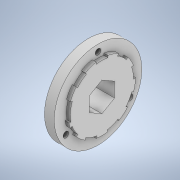
# Autodesk Inventor part: wheel_gearing_mount_short
Saved by Autodesk Inventor 2021 (Build 250183000, 183)
## iProperties
Created: 2021-01-10
Part Number: wheel_gearing_mount_short
Material: Generic
Document SubType Name: Modeling
Designer: Mateusz
Density: 1 g/cm^3
Appearance: Default
Author: Mateusz
Autodesk Inventor part; units mm, degrees
ref_plane "YZ Plane" through (0, 0, 0) normal (1, 0, 0) x (0, 1, 0)
ref_plane "XZ Plane" through (0, 0, 0) normal (0, 1, 0) x (-1, 0, 0)
sketch "Sketch1" plane through (0, 0, 0) normal (1, 0, 0) x (0, 1, 0)
  line L0 (0, 0) -> (7.5, 0)
  line L1 (7.5, 0) -> (3.75, -6.4952)
  line L2 (3.75, -6.4952) -> (-3.75, -6.4952)
  line L3 (-3.75, -6.4952) -> (-7.5, 0)
  line L4 (-7.5, 0) -> (-3.75, 6.4952)
  line L5 (-3.75, 6.4952) -> (3.75, 6.4952)
  line L6 (3.75, 6.4952) -> (7.5, 0)
  circle A0 centre (0, 0) radius 15
  dimension "d0" = 7.5
  dimension "d1" = 30
  constraints: 14 end point, 2 coincident, 1 centre point, 1 horizontal, 13 other
  measures "d0" distance of L0.start L0.end
  measures "d1" diameter of A0
extrude "Extrusion1" add sketch "Sketch1" along normal blind 10.25
sketch "Sketch2" plane through (10.25, 0, 0) normal (1, 0, 0) x (0, 0, -1)
  circle A0 centre (0, 0) radius 22.5
  line L0 (-6.4952, 3.75) -> (0, 7.5) projected
  line L1 (-6.4952, -3.75) -> (-6.4952, 3.75) projected
  line L2 (0, -7.5) -> (-6.4952, -3.75) projected
  line L3 (6.4952, -3.75) -> (0, -7.5) projected
  line L4 (6.4952, 3.75) -> (6.4952, -3.75) projected
  line L5 (0, 7.5) -> (6.4952, 3.75) projected
  dimension "d4" = 45
  constraints: 1 centre point, 1 coincident
  measures "d4" diameter of A0
extrude "Extrusion2" add sketch "Sketch2" against normal blind 5
sketch "Sketch3" plane through (10.25, 0, 0) normal (1, 0, 0) x (0, 0, -1)
  circle A0 centre (0, 19.05) radius 1.45
  circle A1 centre (-16.4978, -9.525) radius 1.45
  circle A2 centre (16.4978, -9.525) radius 1.45
  point P0 (0, 0)
  dimension "d11" = 360
  constraints: 3 centre point, 7 other
extrude "Extrusion3" cut sketch "Sketch3" against normal up to surface (5 mm away)
sketch "Sketch4" plane through (10.25, 0, 0) normal (1, 0, 0) x (0, 0, -1)
  circle A0 centre (0, 19.05) radius 1.45
  line L0 (-3, 17.2409) -> (-3, 16.225)
  line L1 (3, 17.2409) -> (3, 16.225)
  line L2 (13.3804, 11.279) -> (12.7273, 10.5007)
  line L3 (8.7841, 15.1357) -> (8.1311, 14.3574)
  line L4 (17.5, 0.0394) -> (16.4994, -0.137)
  line L5 (16.4581, 5.9483) -> (15.4575, 5.7719)
  line L6 (13.4311, -11.2185) -> (12.5512, -10.7106)
  line L7 (16.4311, -6.0224) -> (15.5512, -5.5144)
  arc A1 (8.7841, 15.1357) -> (3, 17.2409) centre (0, 0) ccw
  arc A2 (16.4311, -6.0224) -> (17.5, 0.0394) centre (0, 0) ccw
  arc A3 (16.4581, 5.9483) -> (13.3804, 11.279) centre (0, 0) ccw
  arc A4 (12.7273, 10.5007) -> (8.1311, 14.3574) centre (0, 0) ccw
  arc A5 (16.4994, -0.137) -> (15.4575, 5.7719) centre (0, 0) ccw
  line L8 (3.0777, -17.2272) -> (2.7302, -16.2726)
  line L9 (3.0777, -17.2272) -> (2.7302, -16.2726)
  line L10 (8.7158, -15.1751) -> (8.3683, -14.2204)
  line L11 (8.7158, -15.1751) -> (8.3683, -14.2204)
  line L12 (-8.7158, -15.1751) -> (-8.3683, -14.2204)
  line L13 (-8.7158, -15.1751) -> (-8.3683, -14.2204)
  line L14 (-3.0777, -17.2272) -> (-2.7302, -16.2726)
  line L15 (-3.0777, -17.2272) -> (-2.7302, -16.2726)
  line L16 (-16.4311, -6.0224) -> (-15.5512, -5.5144)
  line L17 (-16.4311, -6.0224) -> (-15.5512, -5.5144)
  line L18 (-13.4311, -11.2185) -> (-12.5512, -10.7106)
  line L19 (-13.4311, -11.2185) -> (-12.5512, -10.7106)
  arc A6 (8.7158, -15.1751) -> (13.4311, -11.2185) centre (0, 0) ccw
  arc A7 (-13.4311, -11.2185) -> (-8.7158, -15.1751) centre (0, 0) ccw
  arc A8 (-3.0777, -17.2272) -> (3.0777, -17.2272) centre (0, 0) ccw
  arc A9 (12.5512, -10.7106) -> (15.5512, -5.5144) centre (0, 0) ccw
  arc A10 (2.7302, -16.2726) -> (8.3683, -14.2204) centre (0, 0) ccw
  arc A11 (-8.3683, -14.2204) -> (-2.7302, -16.2726) centre (0, 0) ccw
  line L20 (-8.7841, 15.1357) -> (-8.1311, 14.3574)
  line L21 (-13.4115, 11.2412) -> (-12.7273, 10.5007)
  line L22 (-16.4586, 5.9455) -> (-15.4575, 5.7719)
  line L23 (-16.4311, -6.0224) -> (-15.5512, -5.5144)
  line L24 (-13.4311, -11.2185) -> (-12.5512, -10.7106)
  arc A12 (-3, 17.2409) -> (-8.7841, 15.1357) centre (0, 0) ccw
  arc A13 (-13.4115, 11.2412) -> (-15.8894, 7.3321) centre (0, 0) ccw
  arc A14 (-17.2328, -3.0466) -> (-16.4311, -6.0224) centre (0, 0) ccw
  arc A15 (-15.5512, -5.5144) -> (-12.5512, -10.7106) centre (0, 0) ccw
  arc A16 (3, 16.225) -> (-3, 16.225) centre (0, 0) ccw
  arc A17 (-8.1311, 14.3574) -> (-12.7273, 10.5007) centre (0, 0) ccw
  line L25 (-6.4952, 3.75) -> (0, 7.5)
  line L26 (-6.4952, -3.75) -> (-6.4952, 3.75)
  line L27 (0, -7.5) -> (-6.4952, -3.75)
  line L28 (6.4952, -3.75) -> (0, -7.5)
  line L29 (6.4952, 3.75) -> (6.4952, -3.75)
  line L30 (0, 7.5) -> (6.4952, 3.75)
  line L31 (-17.2328, -3.0466) -> (-16.181, -3.229)
  arc A18 (-3, 17.2409) -> (-8.7841, 15.1357) centre (0, 0) ccw
  arc A19 (8.7841, 15.1357) -> (3, 17.2409) centre (0, 0) ccw
  arc A20 (16.4581, 5.9483) -> (13.3804, 11.279) centre (0, 0) ccw
  arc A21 (16.4311, -6.0224) -> (17.5, 0.0394) centre (0, 0) ccw
  arc A22 (8.7158, -15.1751) -> (13.4311, -11.2185) centre (0, 0) ccw
  arc A23 (-3.0777, -17.2272) -> (3.0777, -17.2272) centre (0, 0) ccw
  arc A24 (-13.4311, -11.2185) -> (-8.7158, -15.1751) centre (0, 0) ccw
  arc A25 (-13.4115, 11.2412) -> (-16.4586, 5.9455) centre (0, 0) ccw
  arc A26 (3, 16.225) -> (-3, 16.225) centre (0, 0) ccw
  arc A27 (12.7273, 10.5007) -> (8.1311, 14.3574) centre (0, 0) ccw
  arc A28 (16.4994, -0.137) -> (15.4575, 5.7719) centre (0, 0) ccw
  arc A29 (12.5512, -10.7106) -> (15.5512, -5.5144) centre (0, 0) ccw
  arc A30 (2.7302, -16.2726) -> (8.3683, -14.2204) centre (0, 0) ccw
  arc A31 (-8.3683, -14.2204) -> (-2.7302, -16.2726) centre (0, 0) ccw
  arc A32 (-15.4575, 5.7719) -> (-16.181, -3.229) centre (0, 0) ccw
  arc A33 (-15.5512, -5.5144) -> (-12.5512, -10.7106) centre (0, 0) ccw
  arc A34 (-8.3683, -14.2204) -> (-2.7302, -16.2726) centre (0, 0) ccw
  arc A35 (2.7302, -16.2726) -> (8.3683, -14.2204) centre (0, 0) ccw
  arc A36 (12.5512, -10.7106) -> (15.5512, -5.5144) centre (0, 0) ccw
  arc A37 (16.4994, -0.137) -> (15.4575, 5.7719) centre (0, 0) ccw
  arc A38 (12.7273, 10.5007) -> (8.1311, 14.3574) centre (0, 0) ccw
  arc A39 (3, 16.225) -> (-3, 16.225) centre (0, 0) ccw
  arc A40 (-8.1311, 14.3574) -> (-12.7273, 10.5007) centre (0, 0) ccw
  line L32 (-16.181, -3.229) -> (-17.2328, -3.0466)
  line L33 (-8.7158, -15.1751) -> (-8.3683, -14.2204)
  line L34 (-3.0777, -17.2272) -> (-2.7302, -16.2726)
  line L35 (3.0777, -17.2272) -> (2.7302, -16.2726)
  line L36 (8.3683, -14.2204) -> (8.7158, -15.1751)
  line L37 (12.5512, -10.7106) -> (13.4311, -11.2185)
  line L38 (15.5512, -5.5144) -> (16.4311, -6.0224)
  line L39 (16.4994, -0.137) -> (17.5, 0.0394)
  line L40 (15.4575, 5.7719) -> (16.4581, 5.9483)
  line L41 (12.7273, 10.5007) -> (13.3804, 11.279)
  line L42 (8.1311, 14.3574) -> (8.7841, 15.1357)
  line L43 (3, 16.225) -> (3, 17.2409)
  line L44 (-3, 16.225) -> (-3, 17.2409)
  line L45 (-8.1311, 14.3574) -> (-8.7841, 15.1357)
  line L46 (-12.7273, 10.5007) -> (-13.3804, 11.279)
  line L47 (-12.7273, 10.5007) -> (-13.3804, 11.279)
  line L48 (-15.4575, 5.7719) -> (-16.4586, 5.9455)
  line L49 (-16.181, -3.229) -> (-17.2328, -3.0466)
  line L50 (-16.4311, -6.0224) -> (-15.5512, -5.5144)
  line L51 (-13.4311, -11.2185) -> (-12.5512, -10.7106)
  line L52 (-8.7158, -15.1751) -> (-8.3683, -14.2204)
  line L53 (-3.0777, -17.2272) -> (-2.7302, -16.2726)
  line L54 (3.0777, -17.2272) -> (2.7302, -16.2726)
  point P0 (15.5512, -5.5144)
  point P1 (-8.7158, -15.1751)
  point P2 (-3.0777, -17.2272)
  point P3 (3.0777, -17.2272)
  point P4 (2.7302, -16.2726)
  point P5 (8.7158, -15.1751)
  point P6 (-15.5512, -5.5144)
  point P7 (-2.7302, -16.2726)
  point P8 (-8.3683, -14.2204)
  point P9 (8.3683, -14.2204)
  point P10 (2.7302, -16.2726)
  constraints: 110 end point, 83 point on circle, 41 centre point, 13 collinear, 4 coincident, 3 parallel
ref_plane "Work Plane1" through (12.15, 0, 0) normal (1, 0, 0) x (0, 0, -1)
sketch "Sketch5" plane through (12.15, 0, 0) normal (1, 0, 0) x (0, 0, -1)
  line L0 (6.4952, 3.75) -> (6.4952, -3.75) projected
  circle A0 centre (0, 0) radius 7.5
  constraints: 1 coincident, 3 other
extrude "Extrusion6" add sketch "Sketch4" along normal blind 2 contours L0 A16 L1 A1 L3 A4 L2 A3 L5 A5 L4 A2 L7 A9 L6 A6 L10 A10 L8 A8 L14 A11 L12 A7 L18 A15 L16 A14 L31 A32 L22 A25 A13 L21 A17 L20 A12
sketch "Sketch6" plane through (12.25, 0, 0) normal (1, 0, 0) x (0, 0, -1)
  arc A0 (-13.4115, 11.2412) -> (-16.4586, 5.9455) centre (0, 0) ccw projected
  line L0 (-16.4586, 5.9455) -> (-15.4575, 5.7719) projected
  arc A1 (-15.4575, 5.7719) -> (-16.181, -3.229) centre (0, 0) ccw projected
  line L1 (-16.181, -3.229) -> (-17.2328, -3.0466) projected
  arc A2 (-17.2328, -3.0466) -> (-16.4311, -6.0224) centre (0, 0) ccw projected
  line L2 (-16.4311, -6.0224) -> (-15.5512, -5.5144) projected
  arc A3 (-15.5512, -5.5144) -> (-12.5512, -10.7106) centre (0, 0) ccw projected
  line L3 (-12.5512, -10.7106) -> (-13.4311, -11.2185) projected
  arc A4 (-13.4311, -11.2185) -> (-8.7158, -15.1751) centre (0, 0) ccw projected
  line L4 (-8.7158, -15.1751) -> (-8.3683, -14.2204) projected
  arc A5 (-8.3683, -14.2204) -> (-2.7302, -16.2726) centre (0, 0) ccw projected
  line L5 (-2.7302, -16.2726) -> (-3.0777, -17.2272) projected
  arc A6 (-3.0777, -17.2272) -> (3.0777, -17.2272) centre (0, 0) ccw projected
  line L6 (3.0777, -17.2272) -> (2.7302, -16.2726) projected
  arc A7 (2.7302, -16.2726) -> (8.3683, -14.2204) centre (0, 0) ccw projected
  line L7 (8.3683, -14.2204) -> (8.7158, -15.1751) projected
  arc A8 (8.7158, -15.1751) -> (13.4311, -11.2185) centre (0, 0) ccw projected
  line L8 (13.4311, -11.2185) -> (12.5512, -10.7106) projected
  arc A9 (12.5512, -10.7106) -> (15.5512, -5.5144) centre (0, 0) ccw projected
  line L9 (15.5512, -5.5144) -> (16.4311, -6.0224) projected
  arc A10 (16.4311, -6.0224) -> (17.5, 0.0394) centre (0, 0) ccw projected
  line L10 (17.5, 0.0394) -> (16.4994, -0.137) projected
  arc A11 (16.4994, -0.137) -> (15.4575, 5.7719) centre (0, 0) ccw projected
  line L11 (15.4575, 5.7719) -> (16.4581, 5.9483) projected
  arc A12 (16.4581, 5.9483) -> (13.3804, 11.279) centre (0, 0) ccw projected
  line L12 (13.3804, 11.279) -> (12.7273, 10.5007) projected
  arc A13 (12.7273, 10.5007) -> (8.1311, 14.3574) centre (0, 0) ccw projected
  line L13 (8.1311, 14.3574) -> (8.7841, 15.1357) projected
  arc A14 (8.7841, 15.1357) -> (3, 17.2409) centre (0, 0) ccw projected
  line L14 (3, 17.2409) -> (3, 16.225) projected
  arc A15 (3, 16.225) -> (-3, 16.225) centre (0, 0) ccw projected
  line L15 (-3, 16.225) -> (-3, 17.2409) projected
  arc A16 (-3, 17.2409) -> (-8.7841, 15.1357) centre (0, 0) ccw projected
  line L16 (-8.7841, 15.1357) -> (-8.1311, 14.3574) projected
  arc A17 (-8.1311, 14.3574) -> (-12.7273, 10.5007) centre (0, 0) ccw projected
  line L17 (-12.7273, 10.5007) -> (-13.4115, 11.2412) projected
  line L18 (-6.4952, 3.75) -> (0, 7.5) projected
  line L19 (0, 7.5) -> (6.4952, 3.75) projected
  line L20 (6.4952, 3.75) -> (6.4952, -3.75) projected
  line L21 (6.4952, -3.75) -> (0, -7.5) projected
  line L22 (0, -7.5) -> (-6.4952, -3.75) projected
  line L23 (-6.4952, -3.75) -> (-6.4952, 3.75) projected
  arc A18 (3, 16.225) -> (-3, 16.225) centre (0, 0) ccw projected
  line L24 (3, 16.225) -> (3, 15.9707)
  line L25 (8.1311, 14.3574) -> (7.9676, 14.1626)
  line L26 (12.7273, 10.5007) -> (12.5639, 10.3059)
  line L27 (15.4575, 5.7719) -> (15.2071, 5.7277)
  line L28 (16.4994, -0.137) -> (16.249, -0.1811)
  line L29 (15.5512, -5.5144) -> (16.4311, -6.0224) projected
  line L30 (15.5512, -5.5144) -> (15.331, -5.3873)
  line L31 (12.5512, -10.7106) -> (13.4311, -11.2185) projected
  line L32 (12.5512, -10.7106) -> (12.331, -10.5834)
  line L33 (8.7158, -15.1751) -> (8.3683, -14.2204) projected
  line L34 (8.3683, -14.2204) -> (8.2814, -13.9815)
  line L35 (2.7302, -16.2726) -> (2.6432, -16.0336)
  arc A19 (-8.3683, -14.2204) -> (-2.7302, -16.2726) centre (0, 0) ccw projected
  line L36 (-2.7302, -16.2726) -> (-2.6432, -16.0336)
  line L37 (-8.3683, -14.2204) -> (-8.2814, -13.9815)
  line L38 (-12.5512, -10.7106) -> (-12.331, -10.5834)
  line L39 (-15.5512, -5.5144) -> (-15.331, -5.3873)
  arc A20 (-15.4575, 5.7719) -> (-16.181, -3.229) centre (0, 0) ccw projected
  line L40 (-16.181, -3.229) -> (-15.9166, -3.2749)
  line L41 (-15.4575, 5.7719) -> (-15.2068, 5.7284)
  line L42 (-12.7273, 10.5007) -> (-12.5561, 10.3154)
  line L43 (-8.1311, 14.3574) -> (-7.9676, 14.1626)
  line L44 (-3, 16.225) -> (-3, 15.9707)
  arc A21 (-7.9676, 14.1626) -> (-12.5561, 10.3154) centre (0, 0) ccw
  arc A22 (-15.2068, 5.7284) -> (-15.9166, -3.2749) centre (0, 0) ccw
  arc A23 (-15.331, -5.3873) -> (-12.331, -10.5834) centre (0, 0) ccw
  arc A24 (-8.2814, -13.9815) -> (-2.6432, -16.0336) centre (0, 0) ccw
  arc A25 (2.6432, -16.0336) -> (8.2814, -13.9815) centre (0, 0) ccw
  arc A26 (12.331, -10.5834) -> (15.331, -5.3873) centre (0, 0) ccw
  arc A27 (16.249, -0.1811) -> (15.2071, 5.7277) centre (0, 0) ccw
  arc A28 (12.5639, 10.3059) -> (7.9676, 14.1626) centre (0, 0) ccw
  arc A29 (3, 15.9707) -> (-3, 15.9707) centre (0, 0) ccw
  arc A30 (-3, 16.9871) -> (-8.621, 14.9413) centre (0, 0) ccw
  arc A31 (-13.2408, 11.0564) -> (-16.2089, 5.9022) centre (0, 0) ccw
  arc A32 (-16.9706, -3.092) -> (-16.2113, -5.8955) centre (0, 0) ccw
  arc A33 (-13.2113, -11.0916) -> (-8.629, -14.9366) centre (0, 0) ccw
  arc A34 (-2.9909, -16.9887) -> (2.9909, -16.9887) centre (0, 0) ccw
  arc A35 (8.629, -14.9366) -> (13.2113, -11.0916) centre (0, 0) ccw
  arc A36 (16.2113, -5.8955) -> (17.25, -0.0046) centre (0, 0) ccw
  arc A37 (16.2081, 5.9042) -> (13.2172, 11.0845) centre (0, 0) ccw
  arc A38 (8.621, 14.9413) -> (3, 16.9871) centre (0, 0) ccw
  circle A39 centre (0, 0) radius 17.5
  point P0 (-8.7158, -15.1751)
  point P1 (3.0777, -17.2272)
  point P2 (13.4311, -11.2185)
  point P3 (17.5, 0.0394)
  point P4 (3, 17.2409)
  point P5 (-16.4311, -6.0224)
  point P6 (16.2113, -5.8955)
  point P7 (13.2113, -11.0916)
  point P8 (8.629, -14.9366)
  constraints: 36 end point, 36 point on circle, 18 centre point, 18 point on line, 5 parallel, 3 coincident, 3 collinear, 2 vertical, 3 other
extrude "Extrusion7" cut sketch "Sketch6" against normal up to surface (2 mm away) contours L17 A31 L0 A0 | A39 L16 A17 L17 | L0 A1 L1 A39 | A16 L15 A30 L16 | L1 A32 L2 A2 | A17 L43 A21 L42 | A39 L14 A15 L15 | L41 A22 L40 A1 | L2 A3 L3 A39 | A14 L13 A38 L14 | L3 A33 L4 A4 | A15 L24 A29 L44 | A39 L12 A13 L13 | L39 A23 L38 A3 | L4 A5 L5 A39 | A12 L11 A37 L12 | L5 A34 L6 A6 | A13 L26 A28 L25 | A39 L10 A11 L11 | L37 A24 L36 A5 | L6 A7 L7 A39 | A10 L9 A36 L10 | L7 A35 L8 A8 | A11 L28 A27 L27 | L35 A25 L34 A7 | L8 A9 L9 A39 | A9 L32 A26 L30
body "Solid1"
